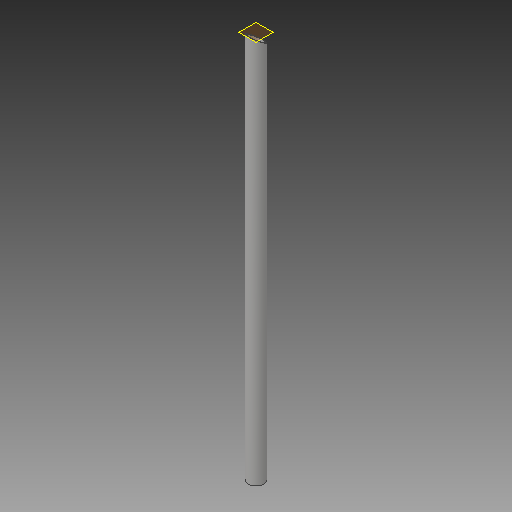
# Autodesk Inventor part: rør
Saved by Autodesk Inventor 2018 (Build 220112000, 112)
## iProperties
Created: 2019-09-25
Part Number: rør
Material: Steel
Document SubType Name: Modeling
Designer: loppen
Density: 7.85 g/cm^3
Appearance: Light Gray
Mass: 4897.75 g
Surface Area: 3339.21 cm^2
Volume: 623.917 cm^3
Author: loppen
Autodesk Inventor part; units mm, degrees
ref_plane "YZ Plane" through (0, 0, 0) normal (1, 0, 0) x (0, 1, 0)
ref_plane "XY Plane" through (0, 0, 0) normal (0, 0, 1) x (1, 0, 0)
sketch "Sketch1" plane through (0, 0, 0) normal (0, 1, 0) x (-1, 0, 0)
  circle A0 centre (0, 0) radius 24.25
  circle A1 centre (0, 0) radius 20.5
  dimension "d0" = 48.5
  dimension "d1" = 3.75
  dimension "d2" = 41
  constraints: 2 centre point, 2 coincident
  measures "d0" diameter of A0
  measures "d1" radial gap between concentric circles of A0 A1
  measures "d2" diameter of A1
extrude "Extrusion1" add sketch "Sketch1" along normal blind 1200
sketch "Sketch2" plane through (0, 0, 0) normal (1, 0, 0) x (0, 1, 0)
  line L0 (0, 24.25) -> (1200, 24.25) projected
  line L1 (0, -24.25) -> (1200, -24.25) projected
  line L2 (1200, 24.25) -> (1166.9155, -24.25)
  line L3 (1200, -24.25) -> (1200, 24.25)
  point P0 (0, 0)
  dimension "d5" = 34.3
  constraints: 4 end point, 1 point on line
  measures "d5" angle of L3 L2
extrude "skrå ende" cut sketch "Sketch2" along normal through all both and the other way through all
ref_plane "Work Plane3" through (0, 1200, 24.25) normal (0, 1, 0) x (-1, 0, 0)
body "Solid1"
